Autodesk Fusion 360 part; units mm, degrees
note: some values were not read from the file. Set by a fixed rule: which sketch regions a step uses.
(part 2 of 3)
  line L839 (23.4221, 53.6514) -> (24.3619, 53.9646)
  arc A136 (20.1531, 55.3381) -> (20.3619, 55.5469) centre (20.1531, 55.5469) ccw
  line L840 (23.2, 56.2) -> (24.8, 56.2)
  line L841 (12.5254, 17.4466) -> (13.0334, 17.4466)
  line L842 (23.1934, 17.4466) -> (23.1934, 17.9546)
  line L843 (16.3619, 55.7558) -> (16.3619, 55.5469)
  line L844 (19.4221, 55.5469) -> (19.4221, 55.7558)
  line L845 (28.2734, 17.9546) -> (27.7654, 17.9546)
  line L846 (17.6054, 17.9546) -> (17.6054, 17.4466)
  line L847 (27.7654, 17.9546) -> (27.7654, 17.4466)
  line L848 (15.5734, 17.9546) -> (15.0654, 17.9546)
  line L849 (20.3619, 53.3381) -> (19.4221, 53.6514)
  arc A137 (28.1531, 55.3381) -> (28.3619, 55.5469) centre (28.1531, 55.5469) ccw
  line L850 (24.3619, 55.7558) -> (24.3619, 55.5469)
  line L851 (7.4221, 53.6514) -> (8.3619, 53.9646)
  arc A138 (27.2, 53.2) -> (28.8, 53.2) centre (28, 54.7) ccw
  line L852 (16.1531, 55.3381) -> (15.6309, 55.3381)
  circle A139 centre (16, 54.7) radius 1.5
  line L853 (8.1531, 55.3381) -> (7.6309, 55.3381)
  line L854 (15.4221, 55.5469) -> (15.4221, 55.7558)
  line L855 (19.2, 56.2) -> (20.8, 56.2)
  line L856 (19.4221, 53.6514) -> (20.3619, 53.9646)
  arc A140 (15.2, 53.2) -> (16.8, 53.2) centre (16, 54.7) ccw
  line L857 (20.6534, 17.9546) -> (20.1454, 17.9546)
  arc A141 (16.1531, 55.3381) -> (16.3619, 55.5469) centre (16.1531, 55.5469) ccw
  line L858 (7.4221, 55.5469) -> (7.4221, 55.7558)
  circle A142 centre (20, 54.7) radius 1.5
  line L859 (8.3619, 55.7558) -> (8.3619, 55.5469)
  arc A143 (19.2, 53.2) -> (20.8, 53.2) centre (20, 54.7) ccw
  line L860 (20.127, 53.8863) -> (20.127, 53.4164)
  arc A144 (15.422, 55.547) -> (15.6309, 55.3381) centre (15.6309, 55.547) ccw
  line L861 (27.4221, 55.5469) -> (27.4221, 55.7558)
  line L862 (8.127, 53.8863) -> (8.127, 53.4164)
  line L863 (14.9863, 12.065) -> (14.9863, 11.43)
  line L864 (32.5438, 12.065) -> (31.9088, 12.065)
  line L865 (25.6381, 11.43) -> (25.8763, 11.43)
  line L866 (30.6388, 11.43) -> (30.6388, 12.065)
  line L867 (16.5738, 9.525) -> (15.9388, 9.525)
  line L868 (36.83, 9.525) -> (36.195, 9.525)
  line L869 (36.9094, 11.43) -> (37.1475, 11.43)
  line L870 (15.9388, 9.525) -> (15.9388, 10.16)
  line L871 (23.9713, 11.43) -> (23.7331, 11.43)
  line L872 (25.8763, 12.065) -> (25.8763, 11.43)
  line L873 (24.9238, 10.16) -> (24.6063, 10.16)
  line L874 (26.7494, 11.43) -> (26.5113, 11.43)
  line L875 (36.195, 11.43) -> (35.8775, 11.43)
  line L876 (25.5587, 10.16) -> (24.9238, 10.16)
  line L877 (25.5587, 9.525) -> (25.5587, 10.16)
  line L878 (24.6063, 11.43) -> (24.6063, 12.065)
  line L879 (31.5913, 9.525) -> (30.9563, 9.525)
  line L880 (15.9388, 10.16) -> (15.6213, 10.16)
  line L881 (16.5738, 10.16) -> (16.8912, 10.16)
  line L882 (15.6213, 11.43) -> (15.6213, 12.065)
  line L883 (26.5113, 11.43) -> (25.8763, 11.43)
  line L884 (24.6063, 11.43) -> (23.9713, 11.43)
  line L885 (37.7825, 11.43) -> (37.7825, 12.065)
  line L886 (17.7644, 11.43) -> (17.5263, 11.43)
  line L887 (35.2425, 11.43) -> (35.0044, 11.43)
  line L888 (15.9388, 11.43) -> (15.6213, 11.43)
  line L889 (24.127, 53.8863) -> (24.127, 53.4164)
  line L890 (27.2, 56.2) -> (28.8, 56.2)
  line L891 (15.6213, 12.065) -> (14.9863, 12.065)
  line L892 (17.5263, 11.43) -> (17.5263, 12.065)
  line L893 (36.195, 9.525) -> (36.195, 10.16)
  line L894 (35.8775, 11.43) -> (35.8775, 12.065)
  line L895 (37.7825, 11.43) -> (37.1475, 11.43)
  line L896 (36.195, 10.16) -> (35.8775, 10.16)
  circle A145 centre (28, 54.7) radius 1.5
  line L897 (38.0206, 11.43) -> (37.7825, 11.43)
  line L898 (35.8775, 11.43) -> (35.2425, 11.43)
  line L899 (24.3619, 53.3381) -> (23.4221, 53.6514)
  line L900 (16.5738, 10.16) -> (15.9388, 10.16)
  line L901 (36.83, 10.16) -> (37.1475, 10.16)
  line L902 (17.5263, 12.065) -> (16.8912, 12.065)
  line L903 (37.7825, 12.065) -> (37.1475, 12.065)
  line L904 (27.4221, 53.6514) -> (28.3619, 53.9646)
  line L905 (37.1475, 12.065) -> (37.1475, 11.43)
  line L906 (15.6213, 11.43) -> (14.9863, 11.43)
  line L907 (36.83, 9.525) -> (36.83, 10.16)
  line L908 (25.5587, 10.16) -> (25.8763, 10.16)
  line L909 (35.2425, 12.065) -> (35.2425, 11.43)
  line L910 (32.5438, 11.43) -> (32.5438, 12.065)
  line L911 (16.8912, 12.065) -> (16.8912, 11.43)
  line L912 (25.5587, 9.525) -> (24.9238, 9.525)
  line L913 (31.9088, 12.065) -> (31.9088, 11.43)
  line L914 (17.5263, 11.43) -> (16.8912, 11.43)
  line L915 (23.9713, 12.065) -> (23.9713, 11.43)
  line L916 (28.1531, 55.3381) -> (27.6309, 55.3381)
  line L917 (28.127, 53.8863) -> (28.127, 53.4164)
  line L918 (16.5738, 9.525) -> (16.5738, 10.16)
  line L919 (35.8775, 12.065) -> (35.2425, 12.065)
  line L920 (36.83, 10.16) -> (36.195, 10.16)
  line L921 (43.6563, 10.16) -> (43.0213, 10.16)
  line L922 (26.5113, 12.065) -> (25.8763, 12.065)
  line L923 (27.2263, 35.475) -> (27.8613, 35.475)
  line L924 (42.0688, 11.43) -> (41.8306, 11.43)
  line L925 (25.8769, 27.4588) -> (26.115, 27.4588)
  line L926 (43.9738, 12.065) -> (43.9738, 11.43)
  line L927 (27.2263, 34.84) -> (27.8613, 34.84)
  line L928 (27.0675, 28.7288) -> (26.75, 28.7288)
  line L929 (43.0213, 10.16) -> (42.7037, 10.16)
  line L930 (24.9238, 9.525) -> (24.9238, 10.16)
  line L931 (30.0038, 12.065) -> (30.0038, 11.43)
  line L932 (30.6388, 11.43) -> (30.0038, 11.43)
  line L933 (38.18, 57.225) -> (38.815, 57.225)
  line L934 (38.815, 57.225) -> (38.815, 56.59)
  line L935 (27.0675, 29.3638) -> (27.0675, 28.7288)
  line L936 (44.6088, 12.065) -> (43.9738, 12.065)
  line L937 (42.7037, 11.43) -> (42.0688, 11.43)
  line L938 (27.8613, 35.475) -> (27.8613, 34.84)
  line L939 (43.0213, 9.525) -> (43.0213, 10.16)
  line L940 (28.655, 27.4588) -> (28.8931, 27.4588)
  line L941 (28.1788, 32.935) -> (28.8138, 32.935)
  line L942 (26.2737, 32.935) -> (26.9088, 32.935)
  line L943 (31.5913, 9.525) -> (31.5913, 10.16)
  line L944 (27.7025, 29.3638) -> (27.7025, 28.7288)
  line L945 (43.7356, 11.43) -> (43.9738, 11.43)
  line L946 (27.0675, 29.3638) -> (27.7025, 29.3638)
  line L947 (30.9563, 10.16) -> (30.6388, 10.16)
  line L948 (31.6706, 11.43) -> (31.9088, 11.43)
  line L949 (42.7037, 12.065) -> (42.0688, 12.065)
  line L950 (28.02, 27.4588) -> (28.02, 26.8238)
  line L951 (28.1788, 33.57) -> (28.8138, 33.57)
  line L952 (24.6063, 12.065) -> (23.9713, 12.065)
  line L953 (27.2263, 34.84) -> (26.9088, 34.84)
  line L954 (31.5913, 10.16) -> (30.9563, 10.16)
  line L955 (38.18, 57.225) -> (38.18, 56.59)
  line L956 (26.9088, 32.935) -> (26.9088, 33.57)
  line L957 (44.6088, 11.43) -> (44.6088, 12.065)
  line L958 (27.1469, 33.57) -> (26.9088, 33.57)
  line L959 (14.9863, 11.43) -> (14.7481, 11.43)
  line L960 (30.0038, 11.43) -> (29.7656, 11.43)
  line L961 (32.7819, 11.43) -> (32.5438, 11.43)
  line L962 (27.8613, 34.84) -> (28.1788, 34.84)
  line L963 (43.0213, 11.43) -> (42.7037, 11.43)
  line L964 (43.6563, 9.525) -> (43.0213, 9.525)
  line L965 (26.75, 26.8238) -> (26.75, 27.4588)
  line L966 (26.9881, 27.4588) -> (26.75, 27.4588)
  line L967 (30.6388, 12.065) -> (30.0038, 12.065)
  line L968 (27.2263, 35.475) -> (27.2263, 34.84)
  line L969 (43.6563, 10.16) -> (43.9738, 10.16)
  line L970 (42.7037, 11.43) -> (42.7037, 12.065)
  line L971 (44.6088, 11.43) -> (43.9738, 11.43)
  line L972 (30.9563, 9.525) -> (30.9563, 10.16)
  line L973 (42.0688, 12.065) -> (42.0688, 11.43)
  line L974 (26.0356, 33.57) -> (26.2737, 33.57)
  line L975 (26.5113, 11.43) -> (26.5113, 12.065)
  line L976 (24.9238, 11.43) -> (24.6063, 11.43)
  line L977 (30.9563, 11.43) -> (30.6388, 11.43)
  line L978 (32.5438, 11.43) -> (31.9088, 11.43)
  line L979 (31.5913, 10.16) -> (31.9088, 10.16)
  line L980 (44.8469, 11.43) -> (44.6088, 11.43)
  line L981 (16.6531, 11.43) -> (16.8912, 11.43)
  line L982 (43.6563, 9.525) -> (43.6563, 10.16)
  line L983 (-4, 19.5263) -> (-8.3, 19.5263)
  line L984 (-8.3, 50.8263) -> (-8.3, 19.5263)
  line L985 (-8.3, 50.8263) -> (49.1, 50.8263)
  line L986 (49.1, 50.8263) -> (49.1, 19.5263)
  line L987 (49.1, 19.5263) -> (44.8, 19.5263)
  line L988 (49, 39.2263) -> (50.1, 39.2263)
  line L989 (50.1, 39.2263) -> (50.1, 31.5263)
  line L990 (0, 1) -> (0, 58.08)
  line L991 (1, 59) -> (52.3, 59)
  line L992 (53.3, 58.08) -> (53.3, 1)
  constraint perpendicular L384 L983
  constraint perpendicular L361 L984
  constraint perpendicular L353 L985
  constraint perpendicular L367 L986
  constraint perpendicular L349 L987
  constraint perpendicular L393 L988
  constraint perpendicular L387 L989
  constraint perpendicular L67 L991
  constraint tangent A1 L992
extrude "Extrude1" add sketch "dxf_import" against normal blind 1.6 contours A0 A1 A2 L0 A5 L116 L118 L119 L120 L121 L124 L125 L127 L130 L133 L134 L137 L138 L139 L140 L141 L146 L151 L154 L155 L158 L161 L162 L164 L168 L169 L171 L173 L174 L176 L177 L178 L180 L183 L187 L206 L221 L297 L298 L299 L302 L303 L312 L314 L316 L317 L328 L330 L332 L333 L340 L341 L342 L347 L351 L353 L354 L356 L357 L358 L359 L362 L363 L364 L365 L367 L368 L370 L371 L372 L373 L375 L378 L380 L382 L386 L387 L388 L390 L391 L392 L393 L552 L579 L580 L589 L590 L601 L718 L719 A88 A90 L725 L728 A93 L729 A97 L752 L754 L760 L762 L763 L767 L769 L770 L771 A102 L774 A105 A106 A107 L777 A111 L780 L781 L783 A115 L786 L787 L788 A118 A119 L800 L801 L985 L986 L987 L988 L989 L990 L991 L992 | L296 L297 L298 L299 L302 L303 L307 L308 L310 L312 L314 L315 L316 L317 L318 L328 L332 L333 L336 L338 L340 L341 L347 L349 L351 L352 L353 L354 L356 L357 L358 L359 L362 L363 L364 L365 L366 L367 L368 L370 L371 L372 L373 L374 L375 L378 L380 L381 L382 L388 L390 L552 L555 L580 L589 L596 L601 L985 L986 L987 L990 | L307 L308 L310 L318 L321 L326 L330 L336 L337 L349 L352 L381 L990 | L336 L338 L343 L349 | L307 L308 L321 L326 L336 L337 L349 | L307 L308 L338 L343 | L0 L118 L119 L718 A97 L788 | L0 L155 L168 L781 L783 A118 | L0 L120 L139 L719 L728 A105 | L0 L178 L206 A119 L800 L801 | L0 L124 L133 A90 L729 L777 | L0 L161 L162 L762 L763 A111 | L0 L121 L140 A88 L725 L787 | L296 L315 L342 L366 L374 L386 L387 L391 L392 L393 L986 L988 L989 | L0 L134 L164 L760 A115 L786 | L0 L174 L183 A93 L752 L754 | L0 L130 L151 L770 L771 A106 | L0 L173 L177 A102 L774 L780 | L0 L154 L169 L767 L769 A107 | L340 L377 L382 L589 L590 L601 L985 | L340 L377 L382 L555 L589 L601 L985 | L341 L373 L552 L579 L580 L985 | L341 L373 L552 L580 L596 L985 | L1 L3 L12 L28 | L2 L4 L51 | L5 L16 L27 L47 | L6 L7 L11 L19 L39 L49 L724 L747 L749 | L7 L9 L13 L50 | L8 L39 L49 L50 L58 | L660 L662 L736 L747 | L11 L48 L52 L54 L58 | L10 L14 L37 L40 | L15 L30 L38 L45 | L17 L24 L41 | L20 L21 L22 L25 L26 L32 L33 L34 L36 L56 L57 L60 L61 L62 L108 L109 L113 L115 L713 L716 L721 L722 L732 L733 L740 L742 L746 L748 L751 L756 L757 L758 | L23 L44 L53 L55 | A7 | A8 | A9 | A11 L72 L78 L84 A29 L96 | L70 A20 L83 L86 | L71 L80 L85 A28 L89 A34 | L76 L77 L88 A36 | L91 L104 L107 | L189 L213 L227 L232 L244 L245 L257 L282 L283 | L227 L229 L235 L252 L256 L270 L273 L293 | L191 L200 L243 L247 L251 L273 L290 L291 | L199 L205 L226 L251 L258 L269 L275 L295 | L225 L226 L230 L259 L271 L272 L276 L294 | L196 L197 L204 L215 L231 L276 L286 L292 | L203 L210 L215 L228 L233 L248 L268 L279 | L190 L192 L195 L203 L278 L280 L281 L284 | A127 | A46 A48 A51 A52 A130 L840 | A142 | A47 A49 A56 A62 L855 A143 | A134 | A50 A53 A57 A65 A126 L835 | A117 | A54 A59 A63 A64 L793 A122 | A139 | A55 A58 A60 A61 L833 A140 | L300 L301 L319 L322 L323 | L306 L311 L313 L327 | A145 | A66 A67 A68 A69 A138 L890 | L397 L400 L402 L442 L450 | L397 L407 L418 L427 L452 | L399 L407 L410 L411 L418 L442 L896 L901 L920 | L403 L404 L410 L427 | L868 L893 L907 L920 | L401 L406 L409 L429 L455 | L409 L412 L413 L414 L419 L451 L880 L881 L900 | L405 L408 L412 L419 L455 | L408 L415 L430 L451 | L867 L870 L900 L918 | A70 | L416 L469 L471 L478 L537 | L422 L436 L471 L484 L519 L539 L927 L953 L962 | L416 L417 L436 L488 L519 | L417 L422 L441 L523 | L923 L927 L938 L968 | L420 L449 L456 L457 L461 L465 L873 L876 L908 | L876 L877 L912 L930 | L439 L453 L457 L468 L472 | L448 L449 L465 L468 L474 | L446 L456 L470 L474 | L421 L425 L460 L463 | L421 L423 L424 L459 L462 L464 L947 L954 L979 | L423 L444 L459 L460 L467 | L447 L454 L462 L467 L475 | L879 L943 L954 L972 | L431 L433 L438 L496 L536 | L437 L438 L473 L515 | L432 L434 L477 L507 L536 | L433 L434 L440 L473 L496 L512 L921 L929 L969 | L921 L939 L964 L982 | A71 | L479 L498 L510 L529 | L509 L525 L526 L529 L538 L540 L609 L631 L928 | L487 L498 L532 L538 L540 | L490 L509 L524 L528 L532 | L609 L935 L944 L946 | L500 L501 L521 L533 | L480 L497 L502 L531 L533 L563 L615 L642 L650 | L497 L500 L502 L542 L558 | L642 L933 L934 L955 | L513 L522 L531 L558 L564 | L481 L492 L493 L581 | L482 L518 L527 L530 | L483 L486 L571 L575 | L485 L511 L553 L588 | L489 L505 L551 L566 | L494 L516 L534 L559 | L495 L499 L541 L570 | L504 L506 L543 L573 | L544 L567 L576 L582 | L545 L547 L591 L597 | L546 L548 L562 L565 | L549 L584 L585 L600 | L550 L587 L592 L599 | L554 L577 L593 L594 | L556 L560 L568 L586 | L557 L574 L578 L583 | L561 L569 L595 L598 | L572 L602 L603 L604 A78 L605 L606 L607 L619 L625 L632 L639 A81 L644 L647 A82 L652 L655 L657 A84 | L619 L633 L638 L639 L654 | L607 L617 L625 L648 L658 | L616 L621 L643 L655 L657 | L634 L645 L647 L652 L656 | A72 A80 | A73 A83 | A74 | A75 | A76 A79 | A77 A85 | L608 L620 L636 L965 | L610 L651 L942 L956 | L612 L613 L618 L623 | L614 L630 L635 L649 | L622 L626 L641 L950 | L628 L653 L941 L951 | L659 L678 L698 L699 | L661 L665 L731 L745 | L663 L667 L677 L697 | L664 L679 L690 L693 | L666 L715 L734 L735 | L668 L682 L686 L706 | L669 L670 L687 L692 | L671 L672 L741 L753 | L673 L674 L694 L708 | L675 L700 L704 L707 | L676 L696 L703 L709 | L680 L691 L695 L702 | L681 L688 L689 L701 | L683 L684 L685 L705 | A86 L710 L768 A113 | L711 A95 L738 A98 | A87 L717 A89 L759 | L720 A94 A96 L775 | L723 L737 L744 L750 | A91 A92 L726 L739 | L727 L755 L761 L778 | A99 L779 A114 L784 | L764 L766 A103 A108 | L765 L772 A104 A112 | A100 L776 L782 A116 | A101 L773 A109 L785 | A110 L790 L802 A124 | L789 L811 L818 L842 | L791 L828 L845 L847 | L792 L817 L824 L848 | L794 A121 L816 A125 | L797 L805 L808 L821 | L798 L804 L810 | L803 L819 L837 L846 | L806 L814 L815 L823 | L807 L812 L822 L841 | L809 L813 L820 L857 | L826 L851 L862 | L829 L830 L832 | L838 L904 L917 | L839 L889 L899 | L849 L856 L860 | L863 L882 L891 L906 | L864 L910 L913 L978 | L866 L931 L932 L967 | L872 L883 L922 L975 | L878 L884 L915 L952 | L885 L895 L903 L905 | L892 L902 L911 L914 | L894 L898 L909 L919 | L926 L936 L957 L971 | L937 L949 L970 L973 makes body 1 in component "PCB"
extrude "Extrude2" add sketch "dxf_import" along normal blind 4.5 and the other way blind 2.3 separate body contours L149 L153 L159 L167 L179 L181 L188 L202 L211 L214 L217 L218 L219 L220 L222 L224 L234 L236 L239 L240 L241 L250 makes body 2 in component "PCB"
extrude "Extrude3" add sketch "dxf_import" against normal blind 2.1 contours L0 L118 L119 L241 | L0 L118 L119 L718 A97 L788 | L0 L155 L168 L781 L783 A118 | L0 L155 L168 L241 | L0 L120 L139 L241 | L0 L120 L139 L719 L728 A105 | L0 L178 L206 A119 L800 L801 | L0 L178 L206 L241 | L0 L124 L133 L241 | L0 L124 L133 A90 L729 L777 | L0 L161 L162 L762 L763 A111 | L0 L161 L162 L241 | L0 L121 L140 L241 | L0 L121 L140 A88 L725 L787 | L0 L134 L164 L760 A115 L786 | L0 L134 L164 L241 | L0 L174 L183 L241 | L0 L174 L183 A93 L752 L754 | L0 L130 L151 L770 L771 A106 | L0 L130 L151 L241 | L0 L173 L177 L241 | L0 L173 L177 A102 L774 L780 | L0 L154 L169 L767 L769 A107 | L0 L154 L169 L241 bodies 1 2 in component "PCB"
extrude "Extrude4" add sketch "dxf_import" along normal blind 13 contours L304 L305 L309 L318 L320 L329 L331 L334 L339 L344 L345 L346 L348 L350 L355 L360 L361 L369 L376 L379 L383 L384 L389 L390 L394 L395 L396 L983 L984 L985 L990 | L296 L297 L298 L299 L302 L303 L307 L308 L310 L312 L314 L315 L316 L317 L318 L328 L332 L333 L336 L338 L340 L341 L347 L349 L351 L352 L353 L354 L356 L357 L358 L359 L362 L363 L364 L365 L366 L367 L368 L370 L371 L372 L373 L374 L375 L378 L380 L381 L382 L388 L390 L552 L555 L580 L589 L596 L601 L985 L986 L987 L990 | L318 L320 L330 L376 L379 L990 | L307 L308 L310 L318 L321 L326 L330 L336 L337 L349 L352 L381 L990 | L336 L338 L343 L349 | L307 L308 L321 L326 L336 L337 L349 | L307 L308 L338 L343 | L296 L315 L342 L366 L374 L386 L387 L391 L392 L393 L986 L988 L989 | L340 L377 L382 L555 L589 L601 L985 | L341 L373 L552 L580 L596 L985 | L1 L3 L12 L28 | L2 L4 L51 | L5 L16 L27 L47 | L10 L14 L37 L40 | L15 L30 L38 L45 | L17 L24 L41 | L20 L21 L22 L25 L26 L32 L33 L34 L36 L56 L57 L60 L61 L62 L108 L109 L113 L115 L713 L716 L721 L722 L732 L733 L740 L742 L746 L748 L751 L756 L757 L758 | L23 L44 L53 L55 | A8 | L300 L301 L319 L322 L323 | L306 L311 L313 L327 | A70 | L416 L469 L471 L478 L537 | L422 L436 L471 L484 L519 L539 L927 L953 L962 | L416 L417 L436 L488 L519 | L417 L422 L441 L523 | L923 L927 L938 L968 | A71 | L479 L498 L510 L529 | L509 L525 L526 L529 L538 L540 L609 L631 L928 | L487 L498 L532 L538 L540 | L490 L509 L524 L528 L532 | L609 L935 L944 L946 | L544 L567 L576 L582 | L545 L547 L591 L597 | L549 L584 L585 L600 | L550 L587 L592 L599 | L557 L574 L578 L583 | L608 L620 L636 L965 | L610 L651 L942 L956 | L622 L626 L641 L950 | L628 L653 L941 L951 | L659 L678 L698 L699 | L663 L667 L677 L697 | L664 L679 L690 L693 | L668 L682 L686 L706 | L669 L670 L687 L692 | L671 L672 L741 L753 | L673 L674 L694 L708 | L675 L700 L704 L707 | L676 L696 L703 L709 | L680 L691 L695 L702 | L681 L688 L689 L701 | L683 L684 L685 L705 | L723 L737 L744 L750 | L727 L755 L761 L778 bodies 1 in component "PCB"
extrude "Extrude5" add sketch "dxf_import" along normal blind 3.3 contours L572 L602 L603 L604 A78 L605 L606 L607 L619 L625 L632 L639 A81 L644 L647 A82 L652 L655 L657 A84 | A72 A80 | A73 A83 | A76 A79 | A77 A85 bodies 1 in component "PCB"
extrude "Extrude6" add sketch "dxf_import" along normal blind 7 contours A74 | A75 bodies 1 in component "PCB"
extrude "Extrude7" add sketch "dxf_import" along normal blind 12.7 contours A127 | A142 | A134 | A117 | A139 | A145 | L798 L804 L810 | L826 L851 L862 | L829 L830 L832 | L838 L904 L917 | L839 L889 L899 | L849 L856 L860 bodies 1 in component "PCB"
extrude "Extrude8" add sketch "dxf_import" along normal blind 0.9 from surface at 12.7 separate body contours A46 A48 A51 A52 A130 L840 | A47 A49 A56 A62 L855 A143 | A50 A53 A57 A65 A126 L835 | A54 A59 A63 A64 L793 A122 | A55 A58 A60 A61 L833 A140 | A66 A67 A68 A69 A138 L890 makes body 3 at (14.6342, 53.6878, 13) makes body 4 at (26.7976, 53.4982, 13) makes body 5 at (12.9432, 56.1143, 13) makes body 6 at (18.3083, 54.8676, 13) makes body 7 at (22.7976, 53.4982, 13) makes body 8 at (9.3658, 53.6878, 13.3) in component "PCB"
extrude "Extrude9" add sketch "dxf_import" along normal blind 5.2 from surface at 12.7 contours A127 | A142 | A134 | A117 | A139 | A145 | L798 L804 L810 | L826 L851 L862 | L829 L830 L832 | L838 L904 L917 | L839 L889 L899 | L849 L856 L860 bodies 1 3 4 5 6 7 8 in component "PCB"
fillet "Fillet1" radius 1.5 6 edges at (26.6015, 54.1576, 17.9) (22.6015, 54.1576, 17.9) (18.6015, 54.1576, 17.9) (14.6015, 54.1576, 17.9) (10.6015, 54.1576, 17.9) (6.6015, 54.1576, 17.9) on bodies 1 in component "PCB"
ref_plane "WorkPlane1" through (26.65, 29.52, 14.5) normal (0, 0, 1) x (1, 0, 0) in component "C64_WiFi2_Top"
ref_plane "WorkPlane1" through (0, 0, -4.6) normal (0, 0, 1) x (1, 0, 0) in component "C64_Wifi2_bottom"
sketch "bottom shell" plane through (0, 0, -4.6) normal (0, 0, 1) x (1, 0, 0) in component "C64_Wifi2_bottom"
  line L0 (1, 59) -> (52.3, 59) construction
  arc A0 (1, 59) -> (0, 58.08) centre (0.96, 58.04) ccw construction
  line L1 (0, 1) -> (0, 58.08) construction
  arc A1 (53.3, 58.08) -> (52.3, 59) centre (52.34, 58.04) ccw construction
  circle A2 centre (49.3, 54.7) radius 1.651 construction
  line L2 (53.3, 58.08) -> (53.3, 1) construction
  arc A3 (52.3, 0) -> (53.3, 1) centre (52.3, 1) ccw construction
  line L3 (1, 0) -> (52.3, 0) construction
  arc A4 (0, 1) -> (1, 0) centre (1, 1) ccw construction
  circle A5 centre (4, 12.8) radius 1.651 construction
  line L4 (-8.3, 50.8263) -> (-8.3, 19.5263) construction
  line L5 (60.92, 0) -> (60.92, -6.8) construction
  line L6 (-7.58, 0) -> (-7.58, -6.8) construction
  line L7 (-8.8, 62.5) -> (60.92, 62.5)
  line L8 (63.92, 59.5) -> (63.92, 3)
  line L9 (60.92, 0) -> (-8.8, 0)
  line L10 (-11.8, 3) -> (-11.8, 59.5)
  arc A6 (60.92, 0) -> (63.92, 3) centre (60.92, 3) ccw
  arc A7 (63.92, 59.5) -> (60.92, 62.5) centre (60.92, 59.5) ccw
  arc A8 (-8.8, 62.5) -> (-11.8, 59.5) centre (-8.8, 59.5) ccw
  arc A9 (-11.8, 3) -> (-8.8, 0) centre (-8.8, 3) ccw
  arc A10 (61.92, 59.5) -> (60.92, 60.5) centre (60.92, 59.5) ccw
  line L11 (-8.8, 60.5) -> (60.92, 60.5)
  arc A11 (-8.8, 60.5) -> (-9.8, 59.5) centre (-8.8, 59.5) ccw
  line L12 (-9.8, 3) -> (-9.8, 59.5)
  arc A12 (-9.8, 3) -> (-8.8, 2) centre (-8.8, 3) ccw
  line L13 (60.92, 2) -> (-8.8, 2)
  arc A13 (60.92, 2) -> (61.92, 3) centre (60.92, 3) ccw
  line L14 (61.92, 59.5) -> (61.92, 3)
  arc A14 (62.72, 59.5) -> (60.92, 61.3) centre (60.92, 59.5) ccw
  line L15 (-8.8, 61.3) -> (60.92, 61.3)
  arc A15 (-8.8, 61.3) -> (-10.6, 59.5) centre (-8.8, 59.5) ccw
  line L16 (-10.6, 3) -> (-10.6, 59.5)
  arc A16 (-10.6, 3) -> (-8.8, 1.2) centre (-8.8, 3) ccw
  arc A17 (60.92, 1.2) -> (62.72, 3) centre (60.92, 3) ccw
  line L17 (62.72, 59.5) -> (62.72, 3)
  line L18 (-0.3, 2) -> (-0.3, 0)
  line L19 (53.5999, 2) -> (53.5999, 0)
  line L20 (60.92, 1.2) -> (53.5999, 1.2)
  line L21 (-0.3, 1.2) -> (-8.8, 1.2)
  circle A18 centre (49.3, 54.7) radius 1.75
  circle A19 centre (4, 12.8) radius 1.75
  circle A20 centre (4, 12.8) radius 3
  circle A21 centre (49.3, 54.7) radius 3
  circle A22 centre (49.3, 54.7) radius 5
  circle A23 centre (4, 12.8) radius 5
  line L22 (49.3, 54.7) -> (0, 54.7) construction
  line L23 (4, 12.8) -> (53.3, 12.8) construction
  line L24 (-2.5, 56.2) -> (1.5, 56.2)
  line L25 (1.5, 56.2) -> (1.5, 53.2)
  line L26 (1.5, 53.2) -> (-2.5, 53.2)
  line L27 (-2.5, 53.2) -> (-2.5, 56.2)
  line L28 (-0.3, 53.2) -> (-0.3, 56.2)
  line L29 (55.8, 11.3) -> (51.8, 11.3)
  line L30 (51.8, 11.3) -> (51.8, 14.3)
  line L31 (51.8, 14.3) -> (55.8, 14.3)
  line L32 (55.8, 14.3) -> (55.8, 11.3)
  line L33 (53.6, 14.3) -> (53.6, 11.3)
  point P0 (-4.2724, 50.8263)
  point P1 (-8.3, 31.6388)
  dimension "d32" = 3
  dimension "d33" = 3
  dimension "d34" = 3.5
  dimension "d35" = 3.5
  dimension "d36" = 2
  dimension "d38" = 0.3
  dimension "d39" = 0.3
  dimension "d40" = 1.2
  dimension "d41" = 3.5
  dimension "d42" = 3.5
  dimension "d43" = 6
  dimension "d44" = 6
  dimension "d45" = 10
  dimension "d46" = 10
  dimension "d49" = 1.5
  dimension "d50" = 3
  dimension "d51" = 2.5
  dimension "d52" = 4
  dimension "d53" = 0.3
  dimension "d54" = 4
  dimension "d55" = 3
  dimension "d56" = 2.5
  dimension "d57" = 1.5
  dimension "d58" = 0.3
  constraint horizontal L7
  constraint vertical L8
  constraint horizontal L9
  constraint vertical L10
  constraint collinear L3 L9
  constraint tangent L8 A6
  constraint tangent L9 A6
  constraint tangent L7 A7
  constraint tangent L8 A7
  constraint equal A6 A7
  constraint tangent L7 A8
  constraint tangent L10 A8
  constraint equal A6 A8
  constraint tangent L9 A9
  constraint tangent L10 A9
  constraint equal A6 A9
  constraint coincident L13 L18.start
  constraint coincident L9 L18.end
  constraint perpendicular L9 L18
  constraint coincident L13 L19.start
  constraint coincident L9 L19.end
  constraint perpendicular L9 L19
  constraint concentric A7 A14
  constraint parallel L7 L15
  constraint concentric A8 A15
  constraint parallel L10 L16
  constraint concentric A9 A16
  constraint parallel L9 L20
  constraint concentric A6 A17
  constraint parallel L8 L17
  constraint tangent A14 L17
  constraint tangent A14 L15
  constraint tangent A17 L17
  constraint tangent L15 A15
  constraint tangent A15 L16
  constraint tangent L16 A16
  constraint tangent A16 L20
  constraint tangent A17 L20
  constraint collinear L20 L21
  constraint coincident L19 L20.end
  constraint coincident L18 L21.start
  constraint concentric A2 A18
  constraint concentric A5 A19
  constraint concentric A19 A20
  constraint concentric A2 A21
  constraint concentric A2 A22
  constraint concentric A19 A23
  constraint coincident A2.centre A18.centre
  constraint coincident L1 L22.end
  constraint perpendicular L1 L22
  constraint coincident A5.centre A19.centre
  constraint coincident L2 L23.end
  constraint perpendicular L2 L23
  constraint horizontal L24
  constraint vertical L25
  constraint horizontal L26
  constraint vertical L27
  constraint coincident L26 L28.start
  constraint coincident L24 L28.end
  constraint perpendicular L24 L28
  constraint horizontal L29
  constraint vertical L30
  constraint horizontal L31
  constraint vertical L32
  constraint coincident L31 L33.start
  constraint coincident L29 L33.end
  constraint perpendicular L29 L33
  measures "d32" radius of A6
  measures "d33" distance of L5 L8
  measures "d34" distance of L0 L7
  measures "d35" distance of L10 P1
  measures "d38" distance of L1 L18
  measures "d40" distance of L7 L15
  measures "d41" diameter of A18
  measures "d42" diameter of A19
  measures "d43" diameter of A20
  measures "d44" diameter of A21
  measures "d45" diameter of A22
  measures "d46" diameter of A23
  measures "d49" distance of L22 L24
  measures "d50" distance of L24.start L26.end
  measures "d51" distance of L1 L27
  measures "d52" distance of L25 L27
  measures "d53" distance of L1 L28
  measures "d54" distance of L30 L32
  measures "d55" distance of L29 L31
  measures "d56" distance of L2 L32
  measures "d57" distance of L23 L31
  measures "d58" distance of L2 L33
extrude "Extrude1'" add sketch "bottom shell" against normal blind 2 separate body contours L7 L8 L9 L10 A6 A7 A8 A9 A14 L15 A15 L16 A16 A17 L17 L18 L19 L20 L21 | L9 L13 L18 L19 | A10 L11 A11 L12 A12 L13 A13 L14 A14 L15 A15 L16 A16 A17 L17 L18 L19 L20 L21 | A10 L11 A11 L12 A12 L13 A13 L14 | A22 | A23 | L24 L26 L27 L28 | L24 L25 L26 L28 | L29 L31 L32 L33 | L29 L30 L31 L33 makes body 9 in component "C64_Wifi2_bottom"
extrude "Extrude2'" add sketch "bottom shell" along normal blind 3 contours A20 | A21 | A22 | A23 | L24 L25 L26 L28 | L29 L30 L31 L33 bodies 9 in component "C64_Wifi2_bottom"
extrude "Extrude3'" add sketch "bottom shell" along normal blind 4.6 contours L24 L26 L27 L28 | L29 L31 L32 L33 bodies 9 in component "C64_Wifi2_bottom"
chamfer "Chamfer1" distance 2 angle 45 2 edges at (44.6384, 52.8919, -1.6) (-0.6616, 10.9919, -1.6) on bodies 9 in component "C64_Wifi2_bottom"
extrude "Extrude4'" add sketch "bottom shell" along normal blind 2 contours L9 L13 L18 L19 bodies 9 in component "C64_Wifi2_bottom"
extrude "Extrude5'" add sketch "bottom shell" along normal blind 10.1 contours A10 L11 A11 L12 A12 L13 A13 L14 A14 L15 A15 L16 A16 A17 L17 L18 L19 L20 L21 bodies 9 in component "C64_Wifi2_bottom"
extrude "Extrude6'" add sketch "bottom shell" along normal blind 9.1 contours L7 L8 L9 L10 A6 A7 A8 A9 A14 L15 A15 L16 A16 A17 L17 L18 L19 L20 L21 bodies 9 in component "C64_Wifi2_bottom"
fillet "Fillet1'" radius 0.5 18 edges at (26.06, 2, -4.6) (61.6271, 2.2929, -4.6) (61.92, 31.25, -4.6) (61.6271, 60.2071, -4.6) (26.06, 60.5, -4.6) (-9.5071, 60.2071, -4.6) (-9.8, 31.25, -4.6) (-9.5071, 2.2929, -4.6) (-0.6616, 14.6081, -4.6) (44.6384, 56.5081, -4.6) (-0.5, 53.2, -4.6) (1.5, 54.7, -4.6) (-0.5, 56.2, -4.6) (-2.5, 54.7, -4.6) (51.8, 12.8, -4.6) (53.8, 11.3, -4.6) (55.8, 12.8, -4.6) (53.8, 14.3, -4.6) on bodies 9 in component "C64_Wifi2_bottom"
fillet "Fillet2" radius 1 8 edges at (-11.8, 31.25, -6.6) (-10.9213, 61.6213, -6.6) (26.06, 62.5, -6.6) (63.0413, 61.6213, -6.6) (63.92, 31.25, -6.6) (63.0413, 0.8787, -6.6) (26.06, 0, -6.6) (-10.9213, 0.8787, -6.6) on bodies 9 in component "C64_Wifi2_bottom"
sketch "top shell" plane through (26.65, 29.52, 14.5) normal (0, 0, 1) x (1, 0, 0) in component "C64_WiFi2_Top"
  line L0 (-35.45, 32.98) -> (34.27, 32.98)
  arc A0 (-35.45, 32.98) -> (-38.45, 29.98) centre (-35.45, 29.98) ccw
  line L1 (-38.45, -26.52) -> (-38.45, 29.98)
  arc A1 (-38.45, -26.52) -> (-35.45, -29.52) centre (-35.45, -26.52) ccw
  line L2 (34.27, -29.52) -> (-35.45, -29.52)
  line L3 (-26.95, -27.52) -> (-26.95, -29.52)
  line L4 (34.27, -27.52) -> (-35.45, -27.52)
  arc A2 (-36.45, -26.52) -> (-35.45, -27.52) centre (-35.45, -26.52) ccw
  line L5 (-36.45, -26.52) -> (-36.45, 29.98)
  arc A3 (-35.45, 30.98) -> (-36.45, 29.98) centre (-35.45, 29.98) ccw
  line L6 (-35.45, 30.98) -> (34.27, 30.98)
  arc A4 (35.27, 29.98) -> (34.27, 30.98) centre (34.27, 29.98) ccw
  line L7 (35.27, 29.98) -> (35.27, -26.52)
  arc A5 (34.27, -27.52) -> (35.27, -26.52) centre (34.27, -26.52) ccw
  arc A6 (34.27, -29.52) -> (37.27, -26.52) centre (34.27, -26.52) ccw
  line L8 (37.27, 29.98) -> (37.27, -26.52)
  arc A7 (37.27, 29.98) -> (34.27, 32.98) centre (34.27, 29.98) ccw
  line L9 (26.9499, -27.52) -> (26.9499, -29.52)
  circle A8 centre (22.65, 25.18) radius 1.651 construction
  circle A9 centre (-22.65, -16.72) radius 1.651 construction
  circle A10 centre (-18.65, 25.18) radius 1.5 construction
  circle A11 centre (-14.65, 25.18) radius 1.5 construction
  circle A12 centre (-10.65, 25.18) radius 1.5 construction
  circle A13 centre (-6.65, 25.18) radius 1.5 construction
  circle A14 centre (-2.65, 25.18) radius 1.5 construction
  circle A15 centre (1.35, 25.18) radius 1.5 construction
  circle A16 centre (22.65, -16.72) radius 1.4 construction
  arc A17 (36.47, 29.98) -> (34.27, 32.18) centre (34.27, 29.98) ccw
  line L10 (-35.45, 32.18) -> (34.27, 32.18)
  arc A18 (-35.45, 32.18) -> (-37.65, 29.98) centre (-35.45, 29.98) ccw
  line L11 (-37.65, -26.52) -> (-37.65, 29.98)
  arc A19 (-37.65, -26.52) -> (-35.45, -28.72) centre (-35.45, -26.52) ccw
  arc A20 (34.27, -28.72) -> (36.47, -26.52) centre (34.27, -26.52) ccw
  line L12 (36.47, 29.98) -> (36.47, -26.52)
  line L13 (34.27, -28.72) -> (26.9499, -28.72)
  line L14 (-26.95, -28.72) -> (-35.45, -28.72)
  circle A21 centre (-18.65, 25.18) radius 1.75
  circle A22 centre (-14.65, 25.18) radius 1.75
  circle A23 centre (-10.65, 25.18) radius 1.75
  circle A24 centre (-6.65, 25.18) radius 1.75
  circle A25 centre (-2.65, 25.18) radius 1.75
  circle A26 centre (1.35, 25.18) radius 1.75
  circle A27 centre (22.65, 25.18) radius 1.25
  circle A28 centre (-22.65, -16.72) radius 1.25
  circle A29 centre (22.65, -16.72) radius 2.5
  line L15 (25.65, -13.72) -> (19.65, -13.72) construction
  line L16 (19.65, -13.72) -> (19.65, -19.72) construction
  line L17 (19.65, -19.72) -> (25.65, -19.72) construction
  line L18 (25.65, -19.72) -> (25.65, -13.72) construction
  line L19 (25.65, -13.72) -> (19.65, -19.72) construction
  line L20 (19.65, -13.72) -> (25.65, -19.72) construction
  line L21 (22.65, -13.72) -> (22.65, -19.72) construction
  line L22 (19.65, -16.72) -> (25.65, -16.72) construction
  line L23 (26, -20.07) -> (19.3, -20.07) construction
  line L24 (19.3, -20.07) -> (19.3, -13.37) construction
  line L25 (19.3, -13.37) -> (26, -13.37) construction
  line L26 (26, -13.37) -> (26, -20.07) construction
  line L27 (26, -20.07) -> (19.3, -13.37) construction
  line L28 (19.3, -20.07) -> (26, -13.37) construction
  line L29 (27, -12.37) -> (18.3, -12.37) construction
  line L30 (18.3, -12.37) -> (18.3, -21.07) construction
  line L31 (18.3, -21.07) -> (27, -21.07) construction
  line L32 (27, -21.07) -> (27, -12.37) construction
  line L33 (27, -12.37) -> (18.3, -21.07) construction
  line L34 (18.3, -12.37) -> (27, -21.07) construction
  line L35 (24.8, -13.37) -> (24.8, -12.37)
  line L36 (26, -14.57) -> (27, -14.57)
  line L37 (20.5, -12.37) -> (20.5, -13.37)
  line L38 (19.3, -14.57) -> (18.3, -14.57)
  line L39 (19.3, -18.87) -> (18.3, -18.87)
  line L40 (20.5, -20.07) -> (20.5, -21.07)
  line L41 (24.8, -20.07) -> (24.8, -21.07)
  line L42 (26, -18.87) -> (27, -18.87)
  line L43 (19.3, -14.57) -> (19.3, -13.37)
  line L44 (19.3, -13.37) -> (20.5, -13.37)
  line L45 (18.3, -12.37) -> (20.5, -12.37)
  line L46 (18.3, -12.37) -> (18.3, -14.57)
  line L47 (24.8, -13.37) -> (26, -13.37)
  line L48 (26, -13.37) -> (26, -14.57)
  line L49 (24.8, -12.37) -> (27, -12.37)
  line L50 (27, -12.37) -> (27, -14.57)
  line L51 (26, -18.87) -> (26, -20.07)
  line L52 (24.8, -20.07) -> (26, -20.07)
  line L53 (24.8, -21.07) -> (27, -21.07)
  line L54 (27, -21.07) -> (27, -18.87)
  line L55 (18.3, -21.07) -> (20.5, -21.07)
  line L56 (20.5, -20.07) -> (19.3, -20.07)
  line L57 (19.3, -20.07) -> (19.3, -18.87)
  line L58 (18.3, -18.87) -> (18.3, -21.07)
  line L59 (26, -15.17) -> (27, -15.17)
  line L60 (27, -15.17) -> (27, -18.27)
  line L61 (27, -18.27) -> (26, -18.27)
  line L62 (26, -18.27) -> (26, -15.17)
  line L63 (18.3, -15.17) -> (19.3, -15.17)
  line L64 (19.3, -15.17) -> (19.3, -18.27)
  line L65 (19.3, -18.27) -> (18.3, -18.27)
  line L66 (18.3, -18.27) -> (18.3, -15.17)
  line L67 (19.3, -18.27) -> (20, -18.27)
  line L68 (20, -18.27) -> (20, -15.17)
  line L69 (20, -15.17) -> (19.3, -15.17)
  line L70 (19.3, -15.17) -> (19.3, -18.27)
  line L71 (26, -18.27) -> (25.3, -18.27)
  line L72 (25.3, -18.27) -> (25.3, -15.17)
  line L73 (25.3, -15.17) -> (26, -15.17)
  line L74 (26, -15.17) -> (26, -18.27)
  circle A30 centre (-22.65, -16.72) radius 3
  circle A31 centre (22.65, 25.18) radius 3
  point P0 (22.65, -16.72)
  point P1 (22.65, -16.72)
  point P2 (22.65, -16.72)
  dimension "d77" = 0.8
  dimension "d78" = 3.5
  dimension "d79" = 3.5
  dimension "d81" = 3.5
  dimension "d82" = 3.5
  dimension "d83" = 3.5
  dimension "d84" = 3.5
  dimension "d85" = 2.5
  dimension "d86" = 2.5
  dimension "d87" = 5
  dimension "d89" = 6
  dimension "d90" = 6
  dimension "d95" = 6.7
  dimension "d96" = 6.7
  dimension "d97" = 8.7
  dimension "d98" = 8.7
  dimension "d99" = 2.2
  dimension "d100" = 2.2
  dimension "d101" = 2.2
  dimension "d102" = 2.2
  dimension "d103" = 2.2
  dimension "d104" = 2.2
  dimension "d105" = 2.2
  dimension "d106" = 2.2
  dimension "d107" = 0.6
  dimension "d108" = 0.6
  dimension "d109" = 0.7
  dimension "d110" = 0.7
  dimension "d117" = 6
  dimension "d118" = 6
  constraint concentric A7 A17
  constraint parallel L0 L10
  constraint concentric A0 A18
  constraint parallel L1 L11
  constraint concentric A1 A19
  constraint parallel L2 L13
  constraint concentric A6 A20
  constraint parallel L8 L12
  constraint tangent A20 L13
  constraint tangent L11 A19
  constraint tangent A17 L12
  constraint tangent A17 L10
  constraint tangent A18 L11
  constraint tangent L10 A18
  constraint tangent A19 L13
  constraint tangent A20 L12
  constraint coincident L9 L13.end
  constraint coincident L3 L14.start
  constraint collinear L13 L14
  constraint concentric A10 A21
  constraint concentric A11 A22
  constraint concentric A12 A23
  constraint concentric A13 A24
  constraint concentric A14 A25
  constraint concentric A15 A26
  constraint concentric A8 A27
  constraint concentric A9 A28
  constraint concentric A16 A29
  constraint perpendicular L15 L16
  constraint parallel L15 L17
  constraint parallel L16 L18
  constraint horizontal L15
  constraint coincident L19 P2
  constraint coincident L20 P2
  constraint coincident P2 P1
  constraint midpoint L15 L21.start
  constraint midpoint L17 L21.end
  constraint midpoint L16 L22.start
  constraint midpoint L18 L22.end
  constraint perpendicular L23 L24
  constraint parallel L23 L25
  constraint parallel L24 L26
  constraint horizontal L23
  constraint coincident L27 P2
  constraint coincident L28 P2
  constraint perpendicular L29 L30
  constraint parallel L29 L31
  constraint parallel L30 L32
  constraint horizontal L29
  constraint coincident L33 P2
  constraint coincident L34 P2
  constraint coincident L25 L35.start
  constraint coincident L29 L35.end
  constraint perpendicular L29 L35
  constraint coincident L26 L36.start
  constraint coincident L32 L36.end
  constraint perpendicular L32 L36
  constraint coincident L29 L37.start
  constraint coincident L25 L37.end
  constraint perpendicular L25 L37
  constraint coincident L24 L38.start
  constraint coincident L30 L38.end
  constraint perpendicular L30 L38
  constraint coincident L24 L39.start
  constraint coincident L30 L39.end
  constraint perpendicular L30 L39
  constraint coincident L23 L40.start
  constraint coincident L31 L40.end
  constraint perpendicular L31 L40
  constraint coincident L31 L41.end
  constraint perpendicular L31 L41
  constraint coincident L26 L42.start
  constraint coincident L32 L42.end
  constraint perpendicular L32 L42
  constraint coincident L28 L25.end
  constraint coincident L25 L26.start
  constraint perpendicular L36 L48
  constraint perpendicular L26 L52
  constraint perpendicular L39 L57
  constraint horizontal L59
  constraint vertical L60
  constraint horizontal L61
  constraint vertical L62
  constraint coincident L32 L60.end
  constraint coincident L26 L59.start
  constraint horizontal L63
  constraint vertical L64
  constraint horizontal L65
  constraint vertical L66
  constraint coincident L24 L64.end
  constraint coincident L30 L63.start
  constraint symmetric L21 L59 L63
  constraint symmetric L21 L61 L65
  constraint horizontal L67
  constraint vertical L68
  constraint horizontal L69
  constraint vertical L70
  constraint horizontal L71
  constraint vertical L72
  constraint horizontal L73
  constraint vertical L74
  constraint concentric A9 A30
  constraint concentric A8 A31
  constraint collinear L63 L69
  constraint collinear L59 L73
  measures "d77" distance of L0 L10
  measures "d78" diameter of A21
  measures "d79" diameter of A22
  measures "d81" diameter of A23
  measures "d82" diameter of A24
  measures "d83" diameter of A25
  measures "d84" diameter of A26
  measures "d85" diameter of A27
  measures "d86" diameter of A28
  measures "d87" diameter of A29
  measures "d89" distance of L16.end L17.end
  measures "d90" distance of L15.end L16.end
  measures "d95" distance of L24.end L25.end
  measures "d96" distance of L23.end L24.end
  measures "d97" distance of L30.end L31.end
  measures "d98" distance of L29.end L30.end
  measures "d99" distance of L32 L35
  measures "d100" distance of L36 L49
  measures "d101" distance of L31 L42
  measures "d102" distance of L41 L54
  measures "d103" distance of L40 L58
  measures "d104" distance of L39 L55
  measures "d105" distance of L38 L45
  measures "d106" distance of L30 L37
  measures "d107" distance of L36 L59
  measures "d108" distance of L42 L61
  measures "d109" distance of L64.end L67.end
  measures "d110" distance of L61.end L71.end
  measures "d117" diameter of A30
  measures "d118" diameter of A31
extrude "Extrude1''" add sketch "top shell" along normal blind 2 separate body contours L0 A0 L1 A1 L2 L3 A6 L8 A7 L9 A17 L10 A18 L11 A19 A20 L12 L13 L14 | L2 L3 L4 L9 | L3 L4 A2 L5 A3 L6 A4 L7 A5 L9 A17 L10 A18 L11 A19 A20 L12 L13 L14 | L4 A2 L5 A3 L6 A4 L7 A5 | A27 | A28 | L35 L36 L47 L48 L49 L50 | L37 L38 L43 L44 L45 L46 | L39 L40 L55 L56 L57 L58 | L41 L42 L51 L52 L53 L54 | L59 L60 L61 L62 L74 | L62 L71 L72 L73 L74 | L63 L64 L65 L66 L70 | L64 L67 L68 L69 L70 | A30 | A31 makes body 10 in component "C64_WiFi2_Top"
extrude "Extrude2''" add sketch "top shell" against normal blind 8.7 contours L3 L4 A2 L5 A3 L6 A4 L7 A5 L9 A17 L10 A18 L11 A19 A20 L12 L13 L14 bodies 10 in component "C64_WiFi2_Top"
extrude "Extrude3''" add sketch "top shell" against normal blind 9.7 contours L0 A0 L1 A1 L2 L3 A6 L8 A7 L9 A17 L10 A18 L11 A19 A20 L12 L13 L14 | L2 L3 L4 L9 bodies 10 in component "C64_WiFi2_Top"
extrude "Extrude4''" add sketch "top shell" against normal blind 14.5 contours A30 | A31 bodies 10 in component "C64_WiFi2_Top"
extrude "Extrude5''" add sketch "top shell" against normal blind 7 contours L35 L36 L47 L48 L49 L50 | L37 L38 L43 L44 L45 L46 | L39 L40 L55 L56 L57 L58 | L41 L42 L51 L52 L53 L54 | L59 L60 L61 L62 L74 | L63 L64 L65 L66 L70 bodies 10 in component "C64_WiFi2_Top"
fillet "Fillet1''" radius 2 8 edges at (63.92, 31.25, 16.5) (63.0413, 61.6213, 16.5) (26.06, 62.5, 16.5) (-10.9213, 61.6213, 16.5) (-11.8, 31.25, 16.5) (-10.9213, 0.8787, 16.5) (26.06, 0, 16.5) (63.0413, 0.8787, 16.5) on bodies 10 in component "C64_WiFi2_Top"
extrude "Extrude6''" add sketch "top shell" against normal blind 1.5 from surface at -5.5 contours L62 L71 L72 L73 L74 | L64 L67 L68 L69 L70 bodies 10 in component "C64_WiFi2_Top"
sketch "frame_hook" plane through (0, 11.25, 0) normal (0, -1, 0) x (1, 0, 0) in component "C64_WiFi2_Top"
  line L0 (53.65, 14.5) -> (52.65, 14.5)
  line L1 (52.65, 14.5) -> (52.65, 9)
  line L2 (52.65, 9) -> (51.95, 9)
  line L3 (51.95, 9) -> (51.95, 7.5)
  line L4 (51.95, 7.5) -> (53.65, 7.5)
  line L5 (53.65, 7.5) -> (53.65, 14.5)
  line L6 (53.65, 7.5) -> (51.95, 7.5)
  line L7 (51.95, 9) -> (51.95, 7.5)
  line L8 (52.65, 9) -> (51.95, 9)
  line L9 (46.65, 7.5) -> (44.95, 7.5)
  line L10 (46.65, 9) -> (46.65, 7.5)
  line L11 (45.95, 9) -> (46.65, 9)
  line L12 (45.95, 9) -> (45.95, 7.5) construction
  line L13 (52.65, 9) -> (52.65, 7.5) construction
  line L14 (46.65, 9) -> (45.95, 7.5)
  line L15 (51.95, 9) -> (52.65, 7.5)
  constraint coincident L11.start L12.start
  constraint coincident L9 L12.end
  constraint perpendicular L9 L12
  constraint coincident L1.end L2.start
  constraint coincident L6 L13.end
  constraint perpendicular L6 L13
  constraint coincident L10.start L11.end
  constraint coincident L12 L14.end
  constraint coincident L2.end L3.start
extrude "Extrude7'" cut sketch "frame_hook" against normal blind 3.5 contours L3 L4 L6 L7 L15 | L9 L10 L14 bodies 10 in component "C64_WiFi2_Top"
chamfer "Chamfer1'" distance 0.2 angle 45 6 edges at (26.3684, 55.3328, 14.5) (22.3684, 55.3328, 14.5) (18.3684, 55.3328, 14.5) (14.3684, 55.3328, 14.5) (10.3684, 55.3328, 14.5) (6.3684, 55.3328, 14.5) on bodies 10 in component "C64_WiFi2_Top"
fillet "Fillet2'" radius 1 21 edges at (61.92, 31.25, 14.5) (61.6271, 2.2929, 14.5) (57.26, 2, 14.5) (-4.55, 2, 14.5) (-9.5071, 2.2929, 14.5) (-9.8, 31.25, 14.5) (-9.5071, 60.2071, 14.5) (26.06, 60.5, 14.5) (61.6271, 60.2071, 14.5) (46.503, 53.6152, 14.5) (1.203, 11.7152, 14.5) (44.95, 9.55, 14.5) (44.95, 12.8, 14.5) (44.95, 16.05, 14.5) (46.05, 17.15, 14.5) (52.55, 17.15, 14.5) (53.65, 16.05, 14.5) (53.65, 12.8, 14.5) (53.65, 9.55, 14.5) (52.55, 8.45, 14.5) (46.05, 8.45, 14.5) on bodies 10 in component "C64_WiFi2_Top"
sketch "plunger" plane through (0, 0, 14.5) normal (0, 0, 1) x (-1, 0, 0) in component "plunger_7mm"
  circle A0 centre (-16, -54.7) radius 1.75
  circle A1 centre (-49.3, -12.8) radius 2.5 construction
  circle A2 centre (-20, -54.7) radius 1.75
  circle A3 centre (-24, -54.7) radius 1.75
  circle A4 centre (-28, -54.7) radius 1.75
  circle A5 centre (-12, -54.7) radius 1.75
  circle A6 centre (-8, -54.7) radius 1.75
  line L0 (-61.92, -3) -> (-61.92, -59.5)
  arc A7 (-61.92, -59.5) -> (-60.92, -60.5) centre (-60.92, -59.5) ccw
  line L1 (-60.92, -60.5) -> (8.8, -60.5)
  arc A8 (8.8, -60.5) -> (9.8, -59.5) centre (8.8, -59.5) ccw
  line L2 (9.8, -59.5) -> (9.8, -3)
  arc A9 (9.8, -3) -> (8.8, -2) centre (8.8, -3) ccw
  line L3 (8.8, -2) -> (-60.92, -2)
  arc A10 (-60.92, -2) -> (-61.92, -3) centre (-60.92, -3) ccw
  line L4 (-52.3, -10.5) -> (-52.3, -15.1) construction
  line L5 (-47, -9.8) -> (-51.6, -9.8)
  line L6 (-46.3, -15.1) -> (-46.3, -10.5) construction
  line L7 (-51.6, -15.8) -> (-47, -15.8)
  line L8 (-52.55, -11.35) -> (-52.05, -11.35) construction
  line L9 (-52.05, -14.25) -> (-52.55, -14.25) construction
  line L10 (-46.55, -14.25) -> (-46.05, -14.25) construction
  line L11 (-46.05, -11.35) -> (-46.55, -11.35) construction
  line L12 (-46.55, -11.35) -> (-46.55, -14.25) construction
  line L13 (-52.05, -11.35) -> (-52.05, -14.25) construction
  circle A11 centre (-49.3, -12.8) radius 2.5 construction
  line L14 (-52.3, -10.95) -> (-51.65, -10.95)
  line L15 (-51.65, -10.95) -> (-51.65, -14.65)
  line L16 (-51.65, -14.65) -> (-52.3, -14.65)
  line L17 (-46.3, -10.95) -> (-46.95, -10.95)
  line L18 (-46.95, -10.95) -> (-46.95, -14.65)
  line L19 (-46.95, -14.65) -> (-46.3, -14.65)
  line L20 (-52.3, -12.8) -> (-46.3, -12.8) construction
  line L21 (-49.3, -9.8) -> (-49.3, -15.8) construction
  line L22 (-52.3, -10.95) -> (-52.3, -10.5) construction
  line L23 (-52.3, -10.5) -> (-52.3, -10.95)
  line L24 (-52.3, -15.1) -> (-52.3, -14.65)
  line L25 (-46.3, -14.65) -> (-46.3, -15.1)
  line L26 (-46.3, -10.5) -> (-46.3, -10.95)
  circle A12 centre (-49.3, -12.8) radius 2.2
  line L27 (-46.3, -10.95) -> (-46.3, -14.65)
  line L28 (-52.3, -10.95) -> (-52.3, -14.65)
  arc A13 (-46.3, -10.5) -> (-47, -9.8) centre (-47, -10.5) ccw
  arc A14 (-51.6, -9.8) -> (-52.3, -10.5) centre (-51.6, -10.5) ccw
  arc A15 (-52.3, -15.1) -> (-51.6, -15.8) centre (-51.6, -15.1) ccw
  arc A16 (-47, -15.8) -> (-46.3, -15.1) centre (-47, -15.1) ccw
  dimension "d132" = 0.4
  dimension "d133" = 0.4
  dimension "d134" = 4.4
  dimension "d139" = 0.7
  dimension "d142" = 0.4
  constraint coincident L4 L14.start
  constraint perpendicular L4 L14
  constraint perpendicular L14 L15
  constraint coincident L4 L16.end
  constraint perpendicular L4 L16
  constraint coincident L6 L17.start
  constraint perpendicular L6 L17
  constraint perpendicular L17 L18
  constraint coincident L6 L19.end
  constraint perpendicular L6 L19
  constraint symmetric L15 L18 L21
  constraint symmetric L16 L19 L21
  constraint symmetric L14 L17 L21
  constraint concentric A11 A12
  constraint coincident L6 L20.end
  constraint coincident L5 L21.start
  constraint tangent L6 A13
  constraint tangent L5 A13
  constraint coincident L4 L20.start
  constraint tangent L5 A14
  constraint tangent L4 A14
  constraint equal A13 A14
  constraint coincident L7 L21.end
  constraint tangent L7 A15
  constraint tangent L4 A15
  constraint equal A13 A15
  constraint tangent L7 A16
  constraint tangent L6 A16
  constraint equal A13 A16
  constraint symmetric L21 L23 L26
  measures "d132" distance of L8 L14
  measures "d133" distance of L13 L15
  measures "d134" diameter of A12
  measures "d139" radius of A13
  measures "d142" distance of L9 L16
extrude "Extrude1'''" add sketch "plunger" along normal blind 3 and the other way blind 0.5 separate body contours A12 makes body 11 in component "plunger_7mm"
extrude "Extrude2'''" add sketch "plunger" against normal blind 4 from surface at -0.5 separate body contours L17 L18 L19 L27 | L14 L15 L16 L28 makes body 12 at (46.3, 12.1833, 12.6667) makes body 13 at (52.3, 12.1833, 12.6667) in component "plunger_7mm"
extrude "Extrude3'''" add sketch "plunger" against normal blind 6.5 from surface at -0.5 contours L5 L7 L14 L15 L16 L17 L18 L19 L23 L24 L25 L26 A13 A14 A15 A16 | A12 bodies 11 12 13 in component "plunger_7mm"